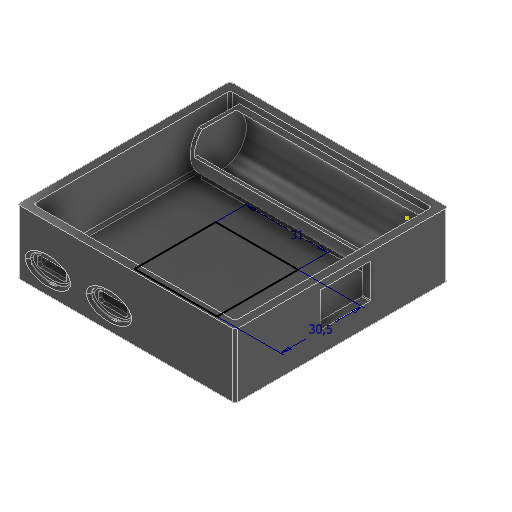
# Autodesk Inventor part: pudelko_v2
Saved by Autodesk Inventor 2026.1 (Build 301233020, 233B)
## iProperties
Created: 2025-08-19
Part Number: pudelko_v2
Material: Generic
Document SubType Name: Modeling
Designer: Paweł
Density: 1 g/cm^3
Appearance: Dark Gray
Mass: 30.7875 g
Surface Area: 279.129 cm^2
Volume: 30.7875 cm^3
Author: Paweł
Autodesk Inventor part; units mm, degrees
ref_plane "YZ Plane" through (0, 0, 0) normal (1, 0, 0) x (0, 1, 0)
ref_plane "XZ Plane" through (0, 0, 0) normal (0, 1, 0) x (-1, 0, 0)
ref_plane "XY Plane" through (0, 0, 0) normal (0, 0, 1) x (1, 0, 0)
sketch "Sketch1" plane through (0, 0, 0) normal (0, 1, 0) x (-1, 0, 0)
  line L0 (77.0121, 67.7143) -> (-2.9879, 67.7143)
  line L1 (-2.9879, 67.7143) -> (-2.9879, -12.2857)
  line L2 (-2.9879, -12.2857) -> (77.0121, -12.2857)
  line L3 (77.0121, -12.2857) -> (77.0121, 67.7143)
  point P0 (0, 0)
  dimension "d0" = 80
  dimension "d1" = 80
  constraints: 8 end point, 2 parallel, 1 horizontal, 1 perpendicular
  measures "d0" distance of L2.end L1.end
  measures "d1" distance of L0.end L1.end
extrude "Extrusion1" add sketch "Sketch1" along normal blind 2
sketch "Sketch2" plane through (0, 2, 0) normal (0, 1, 0) x (1, 0, 0)
  line L0 (2.9879, -67.7143) -> (2.9879, 12.2857) projected
  line L1 (2.9879, 12.2857) -> (-77.0121, 12.2857) projected
  line L2 (-77.0121, 12.2857) -> (-77.0121, -67.7143) projected
  line L3 (-77.0121, -67.7143) -> (2.9879, -67.7143) projected
  line L4 (0.9879, -65.7143) -> (0.9879, 10.2857)
  line L5 (0.9879, 10.2857) -> (-75.0121, 10.2857)
  line L6 (-75.0121, 10.2857) -> (-75.0121, -65.7143)
  line L7 (-75.0121, -65.7143) -> (0.9879, -65.7143)
  point P0 (0, 0)
  dimension "d4" = 2
  constraints: 8 end point, 3 other
  measures "d4" distance between parallel lines of L3 L7
extrude "Extrusion2" add sketch "Sketch2" along normal blind 20
sketch "Sketch4" plane through (-77.0121, 0, 67.7143) normal (0, 0, 1) x (1, 0, 0)
  line L0 (78, 2) -> (2, 2) projected
  line L1 (2, 2) -> (78, 2) projected
  line L2 (2, 2) -> (78, 2) projected
  line L3 (5, 8) -> (16, 8)
  line L4 (5, 4) -> (5, 8)
  line L5 (0, 0) -> (0, 22) projected
  line L6 (0, 0) -> (80, 0) projected
  line L7 (5, 4) -> (16, 4)
  line L8 (16, 4) -> (16, 8)
  point P0 (5, 2)
  dimension "d154" = 11
  dimension "d155" = 4
  dimension "d156" = 5
  dimension "d162" = 2
  constraints: 8 end point, 2 horizontal, 1 perpendicular
  measures "d154" distance of L3.start L3.end
  measures "d155" distance of L4.start L3.start
  measures "d156" distance between parallel lines of L5 L4
  measures "d162" distance between parallel lines of L0 L7
extrude "Extrusion4" cut sketch "Sketch4" against normal up to surface (2 mm away)
sketch "Sketch5" plane through (0.9879, 2, -10.2857) normal (-1, 0, 0) x (0, 0, 1)
  line L0 (76, 0) -> (0, 0) projected
  line L1 (0, 0) -> (0, 20) projected
  circle A0 centre (10, 10) radius 9
  circle A1 centre (10, 10) radius 10
  circle A2 centre (10, 10) radius 10.5
  circle A3 centre (10, 10) radius 9.2
  line L2 (0, 20) -> (76, 20) projected
  line L3 (0, 10) -> (20.5, 10)
  line L4 (13.2016, 0) -> (16.2016, 0)
  line L5 (16.2016, 0) -> (16.2016, 1.5271)
  line L6 (10, 10) -> (10, 20)
  point P0 (10.2857, -2)
  point P1 (78, 0)
  point P2 (10, 0)
  point P3 (13.2016, 0)
  point P4 (13.2016, 20)
  point P5 (6.7984, 20)
  point P6 (0, 13.2016)
  point P7 (0.8, 10)
  point P8 (0, 10)
  point P9 (19.2, 10)
  point P10 (6.7984, 0)
  point P11 (0, 6.7984)
  point P12 (10, 19.2)
  dimension "d11" = 18
  dimension "d12" = 1
  dimension "d13" = 0.5
  dimension "d14" = 0.2
  dimension "d31" = 3
  constraints: 8 end point, 5 point on circle, 4 centre point, 4 midpoint, 4 point on line, 1 horizontal alignment, 1 parallel, 1 perpendicular
  measures "d11" diameter of A0
  measures "d12" radial gap between concentric circles of A0 A1
  measures "d13" radial gap between concentric circles of A1 A2
  measures "d14" radial gap between concentric circles of A0 A3
  measures "d31" distance of L4.start L4.end
extrude "Extrusion5" add sketch "Sketch5" along normal blind 71 contours L0 A2 L5 | L0 A1 L3 A2 | L0 A2 L1 A1 | A1 L3 A3 | L0 L1 A2 | L1 A2 L2 A1 | A1 L6 A3 L3 | L1 L2 A2 picked at (0.4271, 11.4241)
sketch "Sketch10" plane through (0, 2, 0) normal (0, 1, 0) x (1, 0, 0)
  line L0 (-70.0121, -2.9159) -> (-70.0121, -10.2143) projected
  line L1 (-70.0121, 10.2857) -> (-75.0121, 10.2857) projected
  line L2 (-70.0121, -10.2143) -> (-71.5121, -10.2143)
  line L3 (-71.5121, -10.2143) -> (-71.5121, 10.2857)
  line L4 (-71.5121, 10.2857) -> (-70.0121, 10.2857)
  line L5 (-70.0121, 10.2857) -> (-70.0121, -10.2143)
  point P0 (0, 0)
  point P1 (-70.0121, -5.9159)
  dimension "d21" = 1.5
  constraints: 8 end point, 2 parallel, 1 horizontal, 1 perpendicular, 1 point on line
  measures "d21" distance of L3.end L4.end
extrude "Extrusion8" add sketch "Sketch10" along normal up to surface (20 mm away)
sketch "Sketch14" plane through (-70.0121, 2, 10.2143) normal (1, 0, 0) x (0, 0, -1)
  arc A0 (0, 10) -> (4.2984, 1.5271) centre (10.5, 10) ccw projected
  line L0 (0, 0) -> (0, 10) projected
  line L1 (4.2984, 0) -> (0, 0) projected
  line L2 (4.2984, 0) -> (4.2984, 1.5271) projected
  point P0 (10.2143, -2)
extrude "Extrusion11" cut sketch "Sketch14" against normal up to surface (5 mm away)
sketch "Sketch16" plane through (-70.0121, 12, 10.2143) normal (1, 0, 0) x (0, 0, -1)
  arc A0 (1.3, 0) -> (10.5, 9.2) centre (10.5, 0) ccw projected
  arc A1 (0, 0) -> (4.2984, -8.4729) centre (10.5, 0) ccw projected
  circle A2 centre (10.5, 0) radius 10.5
  line L0 (10.5, 10) -> (0, 10) projected
  line L1 (0, 0) -> (0, 10) projected
  point P0 (10.2143, -12)
  point P1 (13.75, -8.6068)
  point P2 (0, 0)
  point P3 (7.2984, 10)
  constraints: 1 centre point, 1 coincident, 1 concentric
extrude "Extrusion13" cut sketch "Sketch16" against normal up to surface (5 mm away) contours L1 L0 A2
sketch "Sketch19" plane through (-70.0121, 22, -0.2857) normal (0, 0, 1) x (1, 0, 0)
  line L0 (71, 0) -> (71, -0.8) projected
  line L1 (71, 0) -> (0, 0) projected
  line L2 (0, -0.8) -> (0, 0) projected
  line L3 (71, -0.8) -> (0, -0.8) projected
  line L4 (71, -0.8) -> (71, -19.2) projected
  line L5 (0, -0.8) -> (71, -0.8)
  line L6 (71, -0.8) -> (71, -2.5024)
  line L7 (71, -2.5024) -> (0, -2.5024)
  line L8 (0, -2.5024) -> (0, -0.8)
  point P0 (70.0121, -22)
  point P1 (71, -10)
  constraints: 8 end point, 2 parallel, 1 horizontal, 1 perpendicular, 1 point on line
extrude "Extrusion15" cut sketch "Sketch19" against normal blind 13
sketch "Sketch20" plane through (0, 22, 0) normal (0, 1, 0) x (1, 0, 0)
  line L0 (-70.0121, 12.2857) -> (-77.0121, 12.2857) projected
  line L1 (-77.0121, 12.2857) -> (2.9879, 12.2857)
  line L2 (2.9879, 12.2857) -> (2.9879, 10.2857)
  line L3 (2.9879, 10.2857) -> (-77.0121, 10.2857)
  line L4 (-77.0121, 10.2857) -> (-77.0121, 12.2857)
  line L5 (2.9879, -67.7143) -> (2.9879, 12.2857) projected
  point P0 (0, 0)
  point P1 (2.9879, 11.2857)
  dimension "d59" = 2
  constraints: 8 end point, 2 parallel, 1 horizontal, 1 midpoint, 1 perpendicular, 1 point on line
  measures "d59" distance of L3.end L0.end
extrude "Extrusion16" cut sketch "Sketch20" against normal through all
sketch "Sketch22" plane through (0, 2, 0) normal (0, 1, 0) x (1, 0, 0)
  line L0 (-75.0121, -65.7143) -> (-75.0121, 10.2857) projected
  line L1 (-71.5121, -5.9159) -> (-71.5121, 10.2857) projected
  line L2 (-75.0121, 10.2857) -> (-71.5121, 10.2857)
  line L3 (-71.5121, 10.2857) -> (-71.5121, 8.2857)
  line L4 (-71.5121, 8.2857) -> (-75.0121, 8.2857)
  line L5 (-75.0121, 8.2857) -> (-75.0121, 10.2857)
  point P0 (0, 0)
  point P1 (-71.5121, 3.5357)
  dimension "d63" = 2
  constraints: 8 end point, 2 parallel, 1 horizontal, 1 perpendicular, 1 point on line
  measures "d63" distance of L2.end L3.end
extrude "Extrusion17" add sketch "Sketch22" along normal up to surface (20 mm away)
sketch "Sketch25" plane through (-70.0121, 19.4976, -5.6173) normal (0, 1, 0) x (1, 0, 0)
  line L0 (71, 4.6684) -> (0, 4.6684) projected
  line L1 (0, -2.0816) -> (0, 3.8684) projected
  line L2 (71, 4.6684) -> (0, 4.6684)
  line L3 (0, 4.6684) -> (0, 2.6684)
  line L4 (0, 2.6684) -> (71, 2.6684)
  line L5 (71, 2.6684) -> (71, 4.6684)
  point P0 (70.0121, -5.6173)
  point P1 (0, 0)
  point P2 (0, 3.8684)
  point P3 (0, -14.5316)
  dimension "d95" = 2
  constraints: 8 end point, 2 parallel, 1 horizontal, 1 perpendicular, 1 point on line
  measures "d95" distance of L3.end L2.end
extrude "Extrusion20" add sketch "Sketch25" along normal up to surface (2.5024 mm away)
sketch "Sketch26" plane through (0, 22, 0) normal (0, 1, 0) x (1, 0, 0)
  line L0 (-71.5121, 8.2857) -> (-75.0121, 8.2857) projected
  line L1 (-72.6308, 8.2857) -> (-68.2243, 8.2857)
  line L2 (-68.2243, 8.2857) -> (-68.2243, -11.3852)
  line L3 (-68.2243, -11.3852) -> (-72.6308, -11.3852)
  line L4 (-72.6308, -11.3852) -> (-72.6308, 8.2857)
  point P0 (0, 0)
  constraints: 8 end point, 2 parallel, 1 horizontal, 1 perpendicular, 1 point on line
extrude "Extrusion21" cut sketch "Sketch26" against normal up to surface (2.5024 mm away)
sketch "Sketch34" plane through (2.9879, 0, -10.2857) normal (0, 0, -1) x (-1, 0, 0)
  point P0 (2.9879, 0)
sketch "Sketch38" plane through (0, 0, 0) normal (0, -1, 0) x (1, 0, 0)
  line L0 (-77.0121, -10.2857) -> (2.9879, -10.2857) projected
  line L1 (2.9879, 67.7143) -> (2.9879, -10.2857) projected
  line L2 (-77.0121, 67.7143) -> (2.9879, 67.7143) projected
  line L3 (-77.0121, -10.2857) -> (-77.0121, 67.7143) projected
  point P0 (0, 0)
extrude "Extrusion31" add sketch "Sketch38" along normal blind 2
sketch "Sketch46" plane through (2.9879, 22, 67.7143) normal (1, 0, 0) x (0, 0, -1)
  line L0 (30.8934, -3) -> (49.8934, -3)
  line L1 (49.8934, -3) -> (49.8934, -16)
  line L2 (49.8934, -16) -> (30.8934, -16)
  line L3 (30.8934, -16) -> (30.8934, -3)
  line L4 (78, -24) -> (0, -24) projected
  point P0 (67.7143, -22)
  dimension "d144" = 13
  dimension "d145" = 19
  dimension "d146" = 8
  constraints: 8 end point, 2 parallel, 1 horizontal, 1 perpendicular
  measures "d144" distance of L2.end L0.start
  measures "d145" distance of L0.start L0.end
  measures "d146" distance between parallel lines of L4 L2
extrude "Extrusion37" cut sketch "Sketch46" against normal up to surface (2 mm away)
fillet "Fillet2" radius 0.3 4 edges at (1.9879, 6, 17.8209) (1.9879, 6, 36.8209) (1.9879, 19, 36.8209) (1.9879, 19, 17.8209)
sketch "Sketch49" plane through (-77.0121, 22, 67.7143) normal (0, 0, 1) x (1, 0, 0)
  line L0 (28, -18) -> (39, -18)
  line L1 (39, -18) -> (39, -14)
  line L2 (39, -14) -> (28, -14)
  line L3 (28, -14) -> (28, -18)
  line L4 (0, -24) -> (0, 0) projected
  line L5 (5.5, -20) -> (2, -20) construction
  line L6 (2, -20) -> (78, -20) construction
  line L7 (78, -20) -> (5.5, -20) construction
  point P0 (77.0121, -22)
  point P1 (16, -14)
  point P2 (16, -18)
  dimension "d163" = 28
  dimension "d164" = 11
  dimension "d165" = 2
  dimension "d166" = 4
  constraints: 8 end point, 2 parallel, 1 horizontal, 1 perpendicular
  measures "d163" distance between parallel lines of L4 L3
  measures "d164" distance of L1.end L2.end
  measures "d165" distance between parallel lines of L6 L0
  measures "d166" distance of L2.end L0.start
extrude "Extrusion40" cut sketch "Sketch49" against normal up to surface (2 mm away)
fillet "Fillet3" radius 1 8 edges at (-72.0121, 4, 66.7143) (-72.0121, 8, 66.7143) (-61.0121, 8, 66.7143) (-61.0121, 4, 66.7143) (-38.0121, 4, 66.7143) (-38.0121, 8, 66.7143) (-49.0121, 8, 66.7143) (-49.0121, 4, 66.7143)
sketch "Sketch51" plane through (-77.0121, 22, -10.2857) normal (-1, 0, 0) x (0, 0, 1)
  arc A0 (16.2016, -18.4729) -> (17.3509, -2.5024) centre (10, -10) ccw projected
  line L0 (0, 0) -> (0, -24) projected
  line L1 (78, -24) -> (0, -24) projected
  line L2 (78, -24) -> (78, 0) projected
  line L3 (0, 0) -> (78, 0) projected
  point P0 (10.2857, -22)
extrude "Extrusion41" add sketch "Sketch51" along normal blind 1
sketch "Sketch52" plane through (2.9879, -2, -10.2857) normal (0, 0, -1) x (-1, 0, 0)
  line L0 (2, 4) -> (74.5, 4) projected
  line L1 (0, 24) -> (81, 24) projected
  line L2 (0, 24) -> (0, 0) projected
  line L3 (0, 0) -> (81, 0) projected
  line L4 (81, 24) -> (81, 0) projected
  point P0 (2.9879, 2)
extrude "Extrusion42" add sketch "Sketch52" along normal blind 1
sketch "Sketch53" plane through (2.9879, -2, 67.7143) normal (1, 0, 0) x (0, 0, -1)
  line L0 (30.8934, 8.3) -> (30.8934, 20.7) projected
  arc A0 (31.1934, 21) -> (30.8934, 20.7) centre (31.1934, 20.7) ccw projected
  line L1 (31.1934, 21) -> (49.5934, 21) projected
  arc A1 (49.8934, 20.7) -> (49.5934, 21) centre (49.5934, 20.7) ccw projected
  line L2 (49.8934, 20.7) -> (49.8934, 8.3) projected
  arc A2 (49.5934, 8) -> (49.8934, 8.3) centre (49.5934, 8.3) ccw projected
  line L3 (49.5934, 8) -> (31.1934, 8) projected
  arc A3 (30.8934, 8.3) -> (31.1934, 8) centre (31.1934, 8.3) ccw projected
  line L4 (0, 24) -> (79, 24) projected
  line L5 (0, 24) -> (0, 0) projected
  line L6 (0, 0) -> (79, 0) projected
  line L7 (79, 24) -> (79, 0) projected
  point P0 (67.7143, 2)
extrude "Extrusion43" add sketch "Sketch53" along normal blind 1
sketch "Sketch54" plane through (-78.0121, -2, 67.7143) normal (0, 0, 1) x (1, 0, 0)
  line L0 (39, 6) -> (30, 6) projected
  arc A0 (29, 7) -> (30, 6) centre (30, 7) ccw projected
  line L1 (29, 7) -> (29, 9) projected
  arc A1 (30, 10) -> (29, 9) centre (30, 9) ccw projected
  line L2 (30, 10) -> (39, 10) projected
  arc A2 (40, 9) -> (39, 10) centre (39, 9) ccw projected
  line L3 (40, 9) -> (40, 7) projected
  arc A3 (39, 6) -> (40, 7) centre (39, 7) ccw projected
  line L4 (16, 6) -> (7, 6) projected
  arc A4 (6, 7) -> (7, 6) centre (7, 7) ccw projected
  line L5 (6, 7) -> (6, 9) projected
  arc A5 (7, 10) -> (6, 9) centre (7, 9) ccw projected
  line L6 (7, 10) -> (16, 10) projected
  arc A6 (17, 9) -> (16, 10) centre (16, 9) ccw projected
  line L7 (17, 9) -> (17, 7) projected
  arc A7 (16, 6) -> (17, 7) centre (16, 7) ccw projected
  line L8 (82, 24) -> (0, 24) projected
  line L9 (0, 0) -> (0, 24) projected
  line L10 (0, 0) -> (82, 0) projected
  line L11 (82, 24) -> (82, 0) projected
  point P0 (78.0121, 2)
extrude "Extrusion44" add sketch "Sketch54" along normal blind 1
sketch "Sketch55" plane through (-78.0121, -2, 68.7143) normal (0, 0, 1) x (1, 0, 0)
  line L0 (82, 0) -> (82, 24) projected
  line L1 (82, 24) -> (0, 24) projected
  line L2 (0, 24) -> (0, 0) projected
  line L3 (0, 0) -> (82, 0) projected
  line L4 (40, 9) -> (40, 7) projected
  arc A0 (39, 6) -> (40, 7) centre (39, 7) ccw projected
  line L5 (39, 6) -> (30, 6) projected
  arc A1 (29, 7) -> (30, 6) centre (30, 7) ccw projected
  line L6 (29, 7) -> (29, 9) projected
  arc A2 (30, 10) -> (29, 9) centre (30, 9) ccw projected
  line L7 (30, 10) -> (39, 10) projected
  arc A3 (40, 9) -> (39, 10) centre (39, 9) ccw projected
  line L8 (17, 9) -> (17, 7) projected
  arc A4 (16, 6) -> (17, 7) centre (16, 7) ccw projected
  line L9 (16, 6) -> (7, 6) projected
  arc A5 (6, 7) -> (7, 6) centre (7, 7) ccw projected
  line L10 (6, 7) -> (6, 9) projected
  arc A6 (7, 10) -> (6, 9) centre (7, 9) ccw projected
  line L11 (7, 10) -> (16, 10) projected
  arc A7 (17, 9) -> (16, 10) centre (16, 9) ccw projected
  ellipse E0 centre (11.5, 8) end of major axis (4, 8) minor radius 4.1418
  line L12 (6, 7) -> (6, 9) projected
  ellipse E1 centre (34.5, 8) end of major axis (27, 8) minor radius 4.1418
  point P0 (78.0121, 2)
  point P1 (11.5, 10)
  point P2 (6, 8)
  point P3 (34.5, 10)
  dimension "d180" = 7.5
  dimension "d181" = 7.5
  dimension "d178" = 2
  dimension "d179" = 5.5
  constraints: 3 midpoint, 1 vertical alignment, 4 other
  measures "d178" distance of point (11.5, 10) point (11.5, 8)
  measures "d179" distance of point (6, 8) point (11.5, 8)
extrude "Extrusion45" cut sketch "Sketch55" against normal blind 1.5 contours E0 | E1
fillet "Fillet4" radius 0.5 2 edges at (-59.0121, 6, 67.2143) (-36.0121, 6, 67.2143)
fillet "Fillet5" radius 0.99 2 edges at (-36.0121, 6, 68.7143) (-59.0121, 6, 68.7143)
fillet "Fillet6" radius 1 7 edges at (-75.0121, 12, 65.7143) (0.9879, 12, 65.7143) (-75.0121, 12, -8.2857) (-78.0121, 10, 68.7143) (-78.0121, 10, -11.2857) (3.9879, 10, -11.2857) (3.9879, 10, 68.7143)
fillet "Fillet7" radius 1 4 edges at (-37.0121, 2, 65.7143) (0.9879, 2, 35.8151) (-73.2621, 2, -8.2857) (-75.0121, 2, 28.7143)
sketch "Sketch56" plane through (0, 22, 0) normal (0, 1, 0) x (1, 0, 0)
  line L0 (-34.8031, -67.7513) -> (-3.8031, -67.7513)
  line L1 (-3.8031, -67.7513) -> (-3.8031, -37.2513)
  line L2 (-3.8031, -37.2513) -> (-34.8031, -37.2513)
  line L3 (-34.8031, -37.2513) -> (-34.8031, -67.7513)
  point P0 (0, 0)
  dimension "d188" = 30.5
  dimension "d189" = 31
  constraints: 8 end point, 2 parallel, 1 horizontal, 1 perpendicular
  measures "d188" distance of L0.end L1.end
  measures "d189" distance of L1.end L2.end
body "Solid1"
